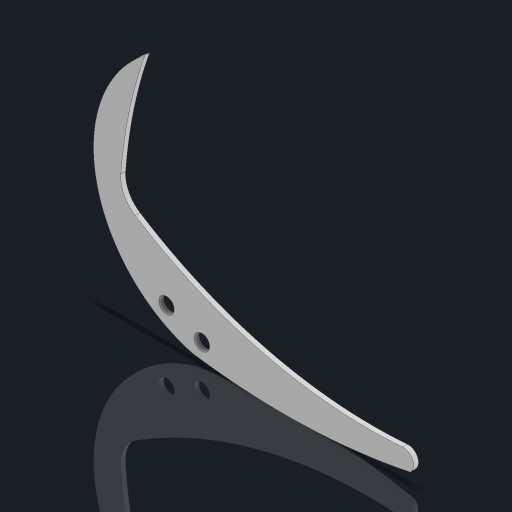
# Autodesk Inventor part: Triball Holder
Saved by Autodesk Inventor 2023.2 (Build 272271030, 271C)
## iProperties
Created: 2024-03-28
Part Number: Triball Holder
Material: Generic
Document SubType Name: Modeling
Designer: Michael
Density: 1 g/cm^3
Appearance: Default
Author: Michael
Autodesk Inventor part; units mm, degrees
ref_plane "YZ Plane" through (0, 0, 0) normal (1, 0, 0) x (0, 1, 0)
ref_plane "XZ Plane" through (0, 0, 0) normal (0, 1, 0) x (-1, 0, 0)
ref_plane "XY Plane" through (0, 0, 0) normal (0, 0, 1) x (1, 0, 0)
ref_plane "Work Plane4" through (0, 0, 1.5875) normal (0, 0, 1) x (1, 0, 0)
sketch "Sketch2" plane through (0, 0, 1.5875) normal (0, 0, 1) x (1, 0, 0)
  arc A0 (-65.0875, -25.4) -> (23.8125, -47.625) centre (12.6658, 96.7006) ccw
  arc A1 (-69.85, -15.875) -> (-65.0875, -25.4) centre (-59.5257, -16.666) ccw
  arc A2 (26.3117, -53.5995) -> (23.8125, -47.625) centre (24.0751, -51.0251) ccw
  arc A3 (-61.9125, 22.225) -> (-69.85, -15.875) centre (81.0518, -27.436) ccw
  arc A4 (-61.9125, 22.225) -> (-46.0375, -55.5625) centre (-34.5823, -12.711) ccw
  arc A5 (-46.0375, -55.5625) -> (26.3117, -53.5995) centre (-15.3756, 148.6013) ccw
  point P0 (0, 0)
  constraints: 12 point on circle, 6 centre point, 3 tangent
extrude "Extrusion2" add sketch "Sketch2" along normal blind 1.5875
sketch "Sketch4" plane through (0, 0, 3.175) normal (0, 0, 1) x (1, 0, 0)
  circle A0 centre (-42.8625, -50.8) radius 2.54
  line L0 (-42.8625, -50.8) -> (-54.6357, -46.0375)
  circle A1 centre (-54.6357, -46.0375) radius 2.54
  point P0 (0, 0)
  dimension "d11" = 5.08
  dimension "d12" = 12.7
  dimension "d13" = 5.08
  constraints: 2 centre point, 2 end point, 1 coincident
  measures "d11" diameter of A0
  measures "d12" distance of L0.start L0.end
  measures "d13" diameter of A1
extrude "Extrusion3" cut sketch "Sketch4" against normal blind 1.5875
body "Solid2"
